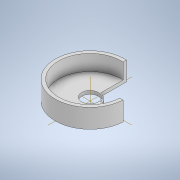
# Autodesk Inventor part: base layer 1
Saved by Autodesk Inventor 2022 (Build 260153000, 153)
## iProperties
Created: 2021-07-05
Part Number: base layer 1
Material: Generic
Document SubType Name: Modeling
Designer: Alicia
Density: 1 g/cm^3
Appearance: Default
Mass: 1.77348 g
Surface Area: 35.637 cm^2
Volume: 1.77348 cm^3
Author: Alicia
Autodesk Inventor part; units mm, degrees
ref_plane "YZ Plane" through (0, 0, 0) normal (1, 0, 0) x (0, 1, 0)
ref_plane "XZ Plane" through (0, 0, 0) normal (0, 1, 0) x (-1, 0, 0)
ref_plane "XY Plane" through (0, 0, 0) normal (0, 0, 1) x (1, 0, 0)
sketch "Sketch9" plane through (0, 0, 0) normal (0, 1, 0) x (-1, 0, 0)
  arc A0 (-1, -20.9762) -> (-20.9762, 1) centre (0, 0) ccw
  line L0 (21, 0) -> (-21, 0) construction
  line L1 (0, 21) -> (0, -21) construction
  line L2 (21, -1) -> (20.9762, -1)
  line L3 (21, 1) -> (20.9762, 1)
  line L4 (-20.9762, 1) -> (-21, 1)
  line L5 (1, 21) -> (1, 20.9762)
  line L6 (1, -20.9762) -> (1, -21)
  line L7 (-1, 21) -> (-1, 20.9762)
  line L8 (-1, -5.9161) -> (-1, -21)
  line L9 (-5.9161, -1) -> (-18.9762, -1)
  circle A1 centre (0, 0) radius 5
  arc A2 (-5.9161, -1) -> (-1, -5.9161) centre (0, 0) ccw
  line L10 (-20.9762, -1) -> (-18.9762, -1)
  line L11 (-19.9762, -1) -> (-19.9762, 1) construction
  line L12 (-19.9762, 1) -> (-20.9762, 1)
  line L13 (-18.9762, 1) -> (-18.9762, -1)
  line L14 (-18.9762, 1) -> (-19.9762, 1)
  point P0 (-4.899, -1)
  point P1 (-1, -4.899)
  point P2 (-20.9762, -1)
  dimension "d30" = 42
  dimension "d35" = 10
  dimension "d48" = 2
  dimension "d49" = 2
  constraints: 30 end point, 8 parallel, 4 perpendicular, 4 point on circle, 3 coincident, 3 point on line, 2 centre point, 1 horizontal, 1 midpoint, 12 other
  measures "d35" diameter of A1
  measures "d48" distance of L9.end L10.start
  measures "d49" distance of L11.start L11.end
extrude "Extrusion5" add sketch "Sketch9" along normal blind 2
chamfer "Chamfer1" distance 0.5 distance2 1 1 edges at (4.2426, 2, -4.2426) measured on face at (14.1627, 2, 6.4351)
sketch "Sketch10" plane through (0, 2, 0) normal (0, 1, 0) x (1, 0, 0)
  arc A0 (1, 20.9762) -> (20.9762, -1) centre (0, 0) ccw
  arc A1 (1, 18.9737) -> (18.9737, -1) centre (0, 0) ccw
  line L0 (20.058, 1) -> (18.9737, 1)
  line L1 (18.9762, 1) -> (5.4083, 1) projected
  line L2 (1, 5.4083) -> (1, 20.9762) projected
  line L3 (1, 18.9737) -> (1, 20.9762)
  line L4 (20.058, 1) -> (20.058, -1) construction
  line L5 (20.058, -1) -> (20.9762, -1)
  line L6 (17.9722, -1) -> (20.9762, -1)
  point P0 (20.9762, 1)
  point P1 (22.9762, 1)
  point P2 (1, 17.9722)
  dimension "d42" = 2
  dimension "d47" = 2
  constraints: 10 end point, 6 point on line, 4 point on circle, 2 centre point, 2 collinear, 1 coincident, 1 perpendicular
  measures "d42" radial gap between concentric circles of A0 A1
  measures "d47" distance of L0.start L4.end
extrude "Extrusion6" add sketch "Sketch10" along normal blind 9.5
body "Solid2"
